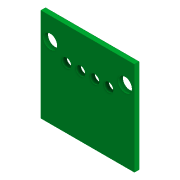
# Autodesk Inventor part: PCB USB-B Hembra
Saved by Autodesk Inventor 2020 (Build 240168000, 168)
## iProperties
Created: 2020-07-11
Part Number: PCB USB-B Hembra
Material: Generic
Document SubType Name: Modeling
Designer: Hernan
Density: 1 g/cm^3
Appearance: Default
Author: Hernan
Autodesk Inventor part; units mm, degrees
ref_plane "YZ Plane" through (0, 0, 0) normal (1, 0, 0) x (0, 1, 0)
ref_plane "XZ Plane" through (0, 0, 0) normal (0, 1, 0) x (-1, 0, 0)
ref_plane "XY Plane" through (0, 0, 0) normal (0, 0, 1) x (1, 0, 0)
sketch "Sketch1" plane through (0, 0, 0) normal (0, 0, 1) x (1, 0, 0)
  line L0 (-19.0052, 9.318) -> (0.9948, 9.318)
  line L1 (0.9948, 9.318) -> (0.9948, -10.682)
  line L2 (0.9948, -10.682) -> (-19.0052, -10.682)
  line L3 (-19.0052, -10.682) -> (-19.0052, 9.318)
  circle A0 centre (-17.0052, 4.5395) radius 1.5
  circle A1 centre (-1.0052, 4.5395) radius 1.5
  dimension "d1" = 20
  dimension "d2" = 20
  dimension "d3" = 3
  dimension "d4" = 2
  constraints: 8 end point, 2 centre point, 2 parallel, 1 horizontal, 1 perpendicular
  measures "d1" distance of L0.start L0.end
  measures "d2" distance of L0.end L1.end
  measures "d3" diameter of A0
  measures "d4" distance from line of A0.centre L3
extrude "Extrusion1" add sketch "Sketch1" along normal blind 1
sketch "Sketch2" plane through (0, 0, 1) normal (0, 0, 1) x (1, 0, 0)
  circle A0 centre (-13.5052, 2.318) radius 1
  circle A1 centre (-10.5052, 2.318) radius 1
  circle A2 centre (-17.0052, 4.5395) radius 1.5 projected
  circle A3 centre (-1.0052, 4.5395) radius 1.5 projected
  line L0 (0.9948, 9.318) -> (-19.0052, 9.318) projected
  line L1 (-9.0052, 9.318) -> (-9.0052, -10.5627)
  circle A4 centre (-4.5052, 2.318) radius 1
  circle A5 centre (-7.5052, 2.318) radius 1
  point P0 (0, 0)
  point P1 (-12.2352, 2.318)
  point P2 (-5.7752, 2.318)
  dimension "d7" = 2
  dimension "d8" = 2
  dimension "d11" = 3
  dimension "d14" = 3.5
  dimension "d19" = 7
  dimension "d21" = 7
  constraints: 4 centre point, 2 end point, 2 symmetric about line, 1 midpoint, 1 vertical, 2 other
  measures "d7" diameter of A0
  measures "d8" diameter of A1
  measures "d11" distance of A1.centre A0.centre
  measures "d14" horizontal distance of A2.centre A0.centre
  measures "d19" distance from line of L0 A1.centre
  measures "d21" distance from line of L0 A0.centre
extrude "Extrusion2" cut sketch "Sketch2" against normal blind 10 contours A0 | A1 | A4 | A5
body "Solid1"
